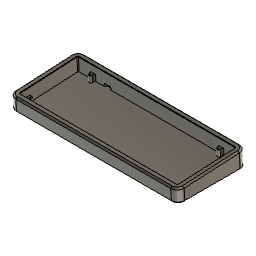
Vault 37 MFR2 (Autodesk Fusion 360 design; units mm, degrees)
Autodesk Fusion 360 part; units mm, degrees
note: some values were not read from the file. Set by a fixed rule: which sketch regions a step uses.
sketch "Outline Sketch" plane through (0, 0, 0) normal (0, 0, 1) x (1, 0, 0)
  line L0 (13.622645, 47.093088) -> (224.322645, 47.093088) construction
  line L1 (224.322645, 47.093088) -> (224.322645, -11.206912) construction
  line L2 (224.322645, -11.206912) -> (195.747645, -11.206912) construction
  line L3 (195.747645, -11.206912) -> (195.747645, -30.256912) construction
  line L4 (195.747645, -30.256912) -> (42.197645, -30.256912) construction
  line L5 (13.622645, 47.093088) -> (13.622645, -11.206912) construction
  line L6 (13.622645, -11.206912) -> (42.197645, -11.206912) construction
  line L7 (42.197645, -30.256912) -> (42.197645, -11.206912) construction
  line L8 (224.622645, -11.506912) -> (196.047645, -11.506912)
  line L9 (196.047645, -11.506912) -> (196.047645, -30.556912)
  line L10 (196.047645, -30.556912) -> (41.897645, -30.556912)
  line L11 (41.897645, -30.556912) -> (41.897645, -11.506912)
  line L12 (13.322645, -11.506912) -> (41.897645, -11.506912)
  line L13 (13.322645, 47.393088) -> (13.322645, -11.506912)
  line L14 (13.322645, 47.393088) -> (224.622645, 47.393088)
  line L15 (224.622645, 47.393088) -> (224.622645, -11.506912)
  line L16 (231.622645, -18.506912) -> (203.047645, -18.506912) construction
  line L17 (203.047645, -18.506912) -> (203.047645, -37.556912) construction
  line L18 (203.047645, -37.556912) -> (34.897645, -37.556912)
  line L19 (34.897645, -37.556912) -> (34.897645, -18.506912) construction
  line L20 (6.322645, -18.506912) -> (34.897645, -18.506912) construction
  line L21 (6.322645, 54.393088) -> (6.322645, -18.506912)
  line L22 (6.322645, 54.393088) -> (231.622645, 54.393088)
  line L23 (231.622645, 54.393088) -> (231.622645, -18.506912)
  line L24 (6.322645, -18.506912) -> (6.322645, -37.556912)
  line L25 (6.322645, -37.556912) -> (34.897645, -37.556912)
  line L26 (203.047645, -37.556912) -> (231.622645, -37.556912)
  line L27 (231.622645, -37.556912) -> (231.622645, -18.506912)
  line L28 (13.322645, -11.506912) -> (13.322645, -34.917536) construction
  line L29 (41.897645, -30.556912) -> (10.561075, -30.556912) construction
  line L30 (13.322645, -11.506912) -> (13.322645, -30.556912)
  line L31 (13.322645, -30.556912) -> (41.897645, -30.556912)
  line L32 (196.047645, -30.556912) -> (224.622645, -30.556912)
  line L33 (224.622645, -11.506912) -> (224.622645, -30.556912)
  dimension "d1" = 210.7
  dimension "d2" = 58.3
  dimension "d3" = 28.575
  dimension "d4" = 19.05
  dimension "d5" = 153.55
  dimension "d6" = 58.3
  dimension "d7" = 28.575
  dimension "d8" = -0.3
  dimension "d9" = -7.3
  constraint horizontal L0
  constraint perpendicular L0 L1
  constraint perpendicular L1 L2
  constraint perpendicular L2 L3
  constraint perpendicular L3 L4
  constraint perpendicular L0 L5
  constraint perpendicular L5 L6
  constraint perpendicular L18 L24
  constraint perpendicular L19 L25
  constraint perpendicular L23 L26
  constraint perpendicular L16 L27
  constraint perpendicular L12 L28
  constraint perpendicular L28 L29
  constraint perpendicular L32 L33
extrude "Extrude1" add sketch "Outline Sketch" along normal blind 18.06
sketch "Angle Sketch" plane through (231.622645, 0, 0) normal (1, 0, 0) x (0, 1, 0)
  line L0 (-37.556912, 0) -> (54.393088, 0)
  line L1 (54.393088, 0) -> (54.393088, 18.06)
  line L2 (54.393088, 18.06) -> (-37.556912, 18.06)
  line L3 (-37.556912, 18.06) -> (-37.556912, 0)
  line L4 (-37.556912, 18.06) -> (-37.556912, -0.215)
  line L5 (-37.556912, -0.215) -> (62.306042, -5.448596)
  line L6 (-37.556912, -0.215) -> (62.443088, -0.215) construction
  dimension "d12" = 18.275
  dimension "d13" = 100
  dimension "d14" = 3
  constraint perpendicular L0 L4
  constraint horizontal L6
  measures "d14" angle of L5 L6
ref_plane "WorkPlane1" through (231.622645, 12.374565, -2.831798) normal (0, -0.052336, -0.99863) x (0, 0.99863, -0.052336)
sketch "Bottom Sketch for Angle" plane through (0, 0, 0) normal (0, 0, -1) x (1, 0, 0)
  line L0 (13.322645, -47.393088) -> (13.322645, 30.556912)
  line L1 (13.322645, 30.556912) -> (224.622645, 30.556912)
  line L2 (224.622645, 30.556912) -> (224.622645, -47.393088)
  line L3 (224.622645, -47.393088) -> (13.322645, -47.393088)
  line L4 (231.622645, 37.556912) -> (6.322645, 37.556912)
  line L5 (6.322645, 37.556912) -> (6.322645, -54.393088)
  line L6 (6.322645, -54.393088) -> (231.622645, -54.393088)
  line L7 (231.622645, -54.393088) -> (231.622645, 37.556912)
  line L8 (231.622645, -54.393088) -> (6.322645, -54.393088)
  line L9 (6.322645, -54.393088) -> (6.322645, 37.556912)
  line L10 (6.322645, 37.556912) -> (231.622645, 37.556912)
  line L11 (231.622645, 37.556912) -> (231.622645, -54.393088)
  constraint horizontal L8
  constraint vertical L9
  constraint horizontal L10
  constraint vertical L11
extrude "Extrude2" add sketch "Bottom Sketch for Angle" along normal up to surface contours L0 L1 L2 L3 | L4 L5 L6 L7 L8 L9 L10 L11 picked at (83.755978, 4.573579) picked at (154.189312, -52.059755) end surface through (231.622645, 12.374565, -2.831798) normal (0, -0.05233596, -0.99862953) offset 0
sketch "USB C Hole Internal Sketch" plane through (0, 47.393088, 0) normal (0, -1, 0) x (1, 0, 0)
  line L0 (13.322645, 0) -> (224.622645, 0)
  line L1 (224.622645, 0) -> (224.622645, 18.06)
  line L2 (224.622645, 18.06) -> (13.322645, 18.06)
  line L3 (13.322645, 18.06) -> (13.322645, 0)
  line L4 (13.322645, 0) -> (52.297645, 0) construction
  line L5 (52.297645, 0) -> (52.297645, 1.83) construction
  line L6 (57.022645, 3.66) -> (47.572645, 3.66)
  line L7 (47.572645, 3.66) -> (47.572645, 0)
  line L8 (47.572645, 0) -> (57.022645, 0)
  line L9 (57.022645, 0) -> (57.022645, 3.66)
  line L10 (57.022645, 3.66) -> (47.572645, 0) construction
  line L11 (47.572645, 3.66) -> (57.022645, 0) construction
  point P0 (52.297645, 1.83)
  dimension "d53" = 38.975
  dimension "d54" = 1.83
  dimension "d55" = 9.45
  dimension "d56" = 3.66
  constraint perpendicular L3 L4
  constraint perpendicular L0 L5
  constraint horizontal L6
  constraint perpendicular L6 L7
  constraint parallel L6 L8
  constraint parallel L7 L9
extrude "Extrude5" cut sketch "USB C Hole Internal Sketch" against normal through all contours L0 L6 L7 L8 L9 picked at (50.722645, 2.44)
fillet "Fillet3" radius 1.55 4 edges at (47.572645, 50.893088, 3.66) (47.572645, 50.893088, 0) (57.022645, 50.893088, 3.66) (57.022645, 50.893088, 0)
sketch "USB C Hole External Sketch" plane through (0, 54.393088, 0) normal (0, 1, 0) x (-1, 0, 0)
  line L0 (-49.122645, 0) -> (-55.472645, 0)
  arc A0 (-57.022645, 1.55) -> (-55.472645, 0) centre (-55.472645, 1.55) ccw
  line L1 (-57.022645, 1.55) -> (-57.022645, 2.11)
  arc A1 (-55.472645, 3.66) -> (-57.022645, 2.11) centre (-55.472645, 2.11) ccw
  line L2 (-55.472645, 3.66) -> (-49.122645, 3.66)
  arc A2 (-47.572645, 2.11) -> (-49.122645, 3.66) centre (-49.122645, 2.11) ccw
  line L3 (-47.572645, 2.11) -> (-47.572645, 1.55)
  arc A3 (-49.122645, 0) -> (-47.572645, 1.55) centre (-49.122645, 1.55) ccw
  line L4 (-6.322645, -5.033895) -> (-6.322645, 18.06)
  line L5 (-6.322645, 18.06) -> (-231.622645, 18.06)
  line L6 (-231.622645, 18.06) -> (-231.622645, -5.033895)
  line L7 (-231.622645, -5.033895) -> (-6.322645, -5.033895)
  line L8 (-45.322645, -2.25) -> (-59.272645, -2.25)
  line L9 (-59.272645, -2.25) -> (-59.272645, 5.91)
  line L10 (-59.272645, 5.91) -> (-45.322645, 5.91)
  line L11 (-45.322645, 5.91) -> (-45.322645, -2.25)
  line L12 (-45.322645, -2.25) -> (-59.272645, 5.91) construction
  line L13 (-59.272645, -2.25) -> (-45.322645, 5.91) construction
  point P0 (-52.297645, 1.83)
  point P1 (-52.297645, 1.83)
  dimension "d60" = 13.95
  dimension "d61" = 8.16
  dimension "d62" = 4.08
  dimension "d63" = 6.975
  constraint horizontal L8
  constraint perpendicular L8 L9
  constraint parallel L8 L10
  constraint parallel L9 L11
extrude "Extrude6" cut sketch "USB C Hole External Sketch" against normal blind 4.549 contours L8 L9 L10 L11 picked at (-51.239312, -1.5)
fillet "Fillet4" radius 3.8 4 edges at (59.272645, 52.118588, -2.25) (59.272645, 52.118588, 5.91) (45.322645, 52.118588, 5.91) (45.322645, 52.118588, -2.25)
chamfer "Chamfer3" distance 0.25 angle 45 8 edges at (58.159651, 54.393088, 4.797006) (59.272645, 54.393088, 1.83) (58.159651, 54.393088, -1.137006) (52.297645, 54.393088, -2.25) (46.435639, 54.393088, -1.137006) (45.322645, 54.393088, 1.83) (46.435639, 54.393088, 4.797006) (52.297645, 54.393088, 5.91)
fillet "Fillet1" radius 9 4 edges at (231.622645, -37.556912, 8.9225) (231.622645, 54.393088, 6.513052) (6.322645, 54.393088, 6.513052) (6.322645, -37.556912, 8.9225)
fillet "Fillet2" radius 1 4 edges at (13.322645, 47.393088, 9.03) (13.322645, -30.556912, 9.03) (224.622645, -30.556912, 9.03) (224.622645, 47.393088, 9.03)
chamfer "Chamfer1" distance 0.5 angle 45 8 edges at (118.972645, 47.393088, 18.06) (224.329752, 47.100195, 18.06) (224.622645, 8.418088, 18.06) (224.329752, -30.264019, 18.06) (118.972645, -30.556912, 18.06) (13.615538, -30.264019, 18.06) (13.322645, 8.418088, 18.06) (13.615538, 47.100195, 18.06)
chamfer "Chamfer2" distance 2 angle 45 16 edges at (118.972645, 54.393088, 18.06) (8.958684, 51.757049, 18.06) (6.322645, 8.418088, 18.06) (8.958684, -34.920873, 18.06) (118.972645, -37.556912, 18.06) (228.986606, -34.920873, 18.06) (231.622645, 8.418088, 18.06) (228.986606, 51.757049, 18.06) (118.972645, 54.393088, -5.033895) (8.958684, 51.757049, -4.895746) (6.322645, 8.418088, -2.624448) (8.958684, -34.920873, -0.353149) (118.972645, -37.556912, -0.215) (228.986606, -34.920873, -0.353149) (231.622645, 8.418088, -2.624448) (228.986606, 51.757049, -4.895746)
sketch "Screw Post Sketch" plane through (0, 0, 0) normal (0, 0, 1) x (-1, 0, 0)
  line L0 (-224.622645, 29.556912) -> (-224.622645, -46.393088)
  arc A0 (-224.622645, -46.393088) -> (-223.622645, -47.393088) centre (-223.622645, -46.393088) ccw
  line L1 (-223.622645, -47.393088) -> (-55.472645, -47.393088)
  arc A1 (-14.322645, -47.393088) -> (-13.322645, -46.393088) centre (-14.322645, -46.393088) ccw
  line L2 (-13.322645, -46.393088) -> (-13.322645, 29.556912)
  line L3 (-14.322645, 30.556912) -> (-223.622645, 30.556912)
  circle A2 centre (-33.247645, -43.993088) radius 2.25
  circle A3 centre (-204.697645, -43.993088) radius 2.25
  line L4 (-35.497645, -43.993088) -> (-35.497645, -46.243088)
  line L5 (-30.997645, -43.993088) -> (-30.997645, -46.243088)
  line L6 (-206.947645, -43.993088) -> (-206.947645, -46.243088)
  line L7 (-202.447645, -43.993088) -> (-202.447645, -46.243088)
  line L8 (-55.472645, -47.393088) -> (-55.472645, -49.844088)
  line L9 (-55.472645, -49.844088) -> (-49.122645, -49.844088)
  line L10 (-49.122645, -49.844088) -> (-49.122645, -47.393088)
  line L11 (-49.122645, -47.393088) -> (-14.322645, -47.393088)
  arc A4 (-30.997645, -46.243088) -> (-29.847645, -47.393088) centre (-29.847645, -46.243088) ccw
  arc A5 (-36.647645, -47.393088) -> (-35.497645, -46.243088) centre (-36.647645, -46.243088) ccw
  line L12 (-29.847645, -47.393088) -> (-36.647645, -47.393088)
  arc A6 (-202.447645, -46.243088) -> (-201.297645, -47.393088) centre (-201.297645, -46.243088) ccw
  arc A7 (-208.097645, -47.393088) -> (-206.947645, -46.243088) centre (-208.097645, -46.243088) ccw
  line L13 (-201.297645, -47.393088) -> (-208.097645, -47.393088)
  circle A8 centre (-63.013265, 29.406912) radius 1.15
  circle A9 centre (-174.932025, 29.406912) radius 1.15
  line L14 (-172.632025, 30.556912) -> (-177.232025, 30.556912)
  arc A10 (-172.632025, 30.556912) -> (-173.782025, 29.406912) centre (-172.632025, 29.406912) ccw
  arc A11 (-176.082025, 29.406912) -> (-177.232025, 30.556912) centre (-177.232025, 29.406912) ccw
  line L15 (-64.163265, 30.556912) -> (-65.313265, 30.556912)
  arc A12 (-60.713265, 30.556912) -> (-61.863265, 29.406912) centre (-60.713265, 29.406912) ccw
  arc A13 (-64.163265, 29.406912) -> (-65.313265, 30.556912) centre (-65.313265, 29.406912) ccw
  arc A14 (-13.322645, 29.556912) -> (-14.322645, 30.556912) centre (-14.322645, 29.556912) ccw
  arc A15 (-223.622645, 30.556912) -> (-224.622645, 29.556912) centre (-223.622645, 29.556912) ccw
  circle A16 centre (-16.463645, 19.865912) radius 2.25
  line L16 (-16.463645, 19.865912) -> (-16.463645, 17.615912) construction
  line L17 (-16.463645, 19.865912) -> (-16.463645, 22.115912) construction
  line L18 (-16.463645, 17.615912) -> (-14.472645, 17.615912)
  line L19 (-16.463645, 22.115912) -> (-14.472645, 22.115912)
  arc A17 (-13.322645, 16.465912) -> (-14.472645, 17.615912) centre (-14.472645, 16.465912) ccw
  arc A18 (-14.472645, 22.115912) -> (-13.322645, 23.265912) centre (-14.472645, 23.265912) ccw
  line L20 (-13.322645, 23.265912) -> (-13.322645, 16.465912)
  circle A19 centre (-221.481645, 19.865912) radius 2.25
  line L21 (-221.48246, 17.615912) -> (-223.463577, 17.61663)
  line L22 (-221.48083, 22.115912) -> (-223.481745, 22.116637)
  arc A20 (-224.631327, 23.268229) -> (-223.481745, 22.116637) centre (-223.481328, 23.266636) ccw
  line L23 (-224.613994, 16.467625) -> (-224.631327, 23.268229)
  arc A21 (-223.463577, 17.61663) -> (-224.613994, 16.467625) centre (-223.463994, 16.46663) ccw
  line L24 (-224.62266, 19.867927) -> (-223.731641, 19.870198) construction
  line L25 (-223.731641, 19.870198) -> (-221.481645, 19.865912)
  point P0 (-35.497645, -47.393088)
  point P1 (-30.997645, -47.393088)
  point P2 (-206.947645, -47.393088)
  point P3 (-202.447645, -47.393088)
  point P4 (-173.782025, 30.556912)
  point P5 (-176.082025, 30.556912)
  point P6 (-61.863265, 30.556912)
  point P7 (-60.713265, 30.556912)
  point P8 (-13.322645, 17.615912)
  point P9 (-13.322645, 22.115912)
  dimension "d27" = 4.5
  dimension "d28" = 4.5
  dimension "d31" = 3.4
  dimension "d32" = 3.4
  dimension "d33" = 19.925
  dimension "d34" = 19.925
  dimension "d71" = 1.15
  dimension "d72" = 1.15
  dimension "d75" = 1.15
  dimension "d76" = 1.15
  dimension "d86" = 2.3
  dimension "d88" = 2.3
  dimension "d90" = 1.15
  dimension "d91" = 1.15
  dimension "d92" = 1.15
  dimension "d93" = 1.15
  dimension "d94" = 1.15
  dimension "d95" = 1.15
  dimension "d96" = 1.15
  dimension "d97" = 1.15
  dimension "d98" = 1.15
  dimension "d99" = 1.15
  dimension "d100" = 4.5
  dimension "d101" = 3.141
  dimension "d102" = 10.691
  dimension "d104" = 1.15
  dimension "d106" = 1.15
  dimension "d107" = 4.5
  dimension "d108" = 1.15
  dimension "d109" = 1.15
  dimension "d110" = 3.141
  dimension "d111" = 3.141
  dimension "d112" = 0.891019
  dimension "d113" = 2.25
  dimension "d114" = 10.691
  constraint tangent A2 L4
  constraint perpendicular L1 L4
  constraint tangent A2 L5
  constraint perpendicular L1 L5
  constraint tangent A3 L6
  constraint perpendicular L1 L6
  constraint tangent A3 L7
  constraint perpendicular L1 L7
  constraint tangent L5 A4
  constraint tangent L4 A5
  constraint tangent A5 L12
  constraint tangent L7 A6
  constraint tangent L6 A7
  constraint tangent A7 L13
  constraint parallel L2 L16
  constraint parallel L16 L17
  constraint tangent A16 L18
  constraint tangent A16 L19
  constraint tangent L18 A17
  constraint tangent L19 A18
  constraint tangent A19 L22
  constraint tangent A19 L21
  constraint tangent L22 A20
  constraint tangent L21 A21
  constraint parallel L21 L22
  constraint perpendicular L23 L24
  measures "d27" diameter of A2
  measures "d28" diameter of A3
  measures "d71" radius of A4
  measures "d72" radius of A5
  measures "d75" radius of A6
  measures "d76" radius of A7
  measures "d86" diameter of A8
  measures "d88" diameter of A9
  measures "d94" radius of A10
  measures "d95" radius of A11
  measures "d98" radius of A12
  measures "d99" radius of A13
  measures "d100" diameter of A16
  measures "d104" radius of A17
  measures "d106" radius of A18
  measures "d107" diameter of A19
  measures "d108" radius of A20
  measures "d109" radius of A21
extrude "Extrude4" add sketch "Screw Post Sketch" along normal blind 8.41 contours L0 A19 L21 L22 A20 L23 A21 | L3 A9 L14 A11 | A19 | L3 A9 L14 A10 | A9 | L1 A3 L6 L7 A6 A7 L13 | L3 A8 L15 A13 | A8 | A3 | L3 A8 A12 | A2 L4 L5 L11 A4 A5 L12 | L2 A16 L18 L19 A17 A18 L20 | A2 | A16 picked at (-224.086834, 20.989945) picked at (-176.047384, 29.980646) picked at (-220.951935, 19.898635) picked at (-173.816666, 29.980646) picked at (-174.932025, 29.042801) picked at (-204.641598, -46.820399) picked at (-64.163265, 30.204737) picked at (-62.960015, 29.04416) picked at (-204.641598, -45.585971) picked at (-61.897906, 29.980646) picked at (-33.303693, -46.820399) picked at (-13.741351, 19.865912) picked at (-33.685339, -44.503218) picked at (-17.029108, 21.275341)
hole "Hole1" at (33.247645, 43.993088, 8.41) direction (0, 0, -1) diameter 1.8 depth 4 tip angle 180
hole "Hole2" at (204.697645, 43.993088, 8.41) direction (0, 0, -1) diameter 1.8 depth 4 tip angle 180
hole "Hole3" at (221.481645, -19.865912, 8.41) direction (0, 0, -1) diameter 1.8 depth 4 tip angle 180
hole "Hole4" at (16.463645, -19.865912, 8.41) direction (0, 0, -1) diameter 1.8 depth 4 tip angle 180
extrude "Extrude3" add 1 faces at (153.522645, 23.077335, -3.392706) along direction (0, 0.05233596, 0.99862953) blind 1
move_body "Move1" bodies 1 to x (1, 0, 0) y (0, 0.99862953, 0.05233596) z (0, -0.05233596, 0.99862953) at (0, 0.041949, 1.968023)
equation "d39 = 7.9 mm + 0.51 mm"
equation "d53 = 0.875 mm + 19.05 mm * 2"
equation "d54 = ( 3.66 / 2 ) * 1 mm"
equation "d55 = ( 4.725 * 2 ) * 1 mm"
equation "d62 = d61 / 2"
equation "d63 = d60 / 2"
equation "d64 = -3.5 mm - 1.049 mm"
equation "d90 = ( 2.3 / 2 ) * 1 mm"
equation "d91 = ( 2.3 / 2 ) * 1 mm"
